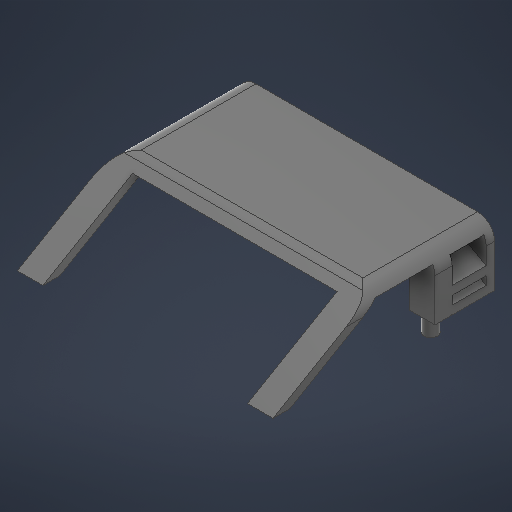
# Autodesk Inventor part: dach
Saved by Autodesk Inventor 2026.2 (Build 302298000, 298)
## iProperties
Created: 2026-08-16
Part Number: dach
Material: Tworzywo sztuczne ABS
Document SubType Name: Modeling
Designer: wojsl
Density: 1.06 g/cm^3
Appearance: Gładki — biały
Author: wojsl
Autodesk Inventor part; units mm, degrees
ref_plane "YZ Plane" through (0, 0, 0) normal (1, 0, 0) x (0, 1, 0)
ref_plane "XZ Plane" through (0, 0, 0) normal (0, 1, 0) x (-1, 0, 0)
ref_plane "XY Plane" through (0, 0, 0) normal (0, 0, 1) x (1, 0, 0)
sketch "Szkic1" plane through (0, 0, 0) normal (0, 0, 1) x (1, 0, 0)
  line L0 (-10.8101, 8.1046) -> (-12.3101, 8.1046)
  line L1 (-12.3101, 8.1046) -> (-12.3101, 11.6046)
  line L2 (-12.3101, 11.6046) -> (-10.8101, 11.6046)
  line L3 (-10.8101, 11.6046) -> (-10.8101, 8.1046)
  line L4 (-10.8101, 11.6046) -> (1.1899, 11.6046)
  line L5 (1.1899, 11.6046) -> (1.1899, 11.1716)
  line L6 (1.1899, 11.1716) -> (-10.8101, 11.1716)
  line L7 (-10.8101, 11.1716) -> (-10.8101, 11.6046)
  line L8 (1.1899, 11.6046) -> (2.6899, 11.6046)
  line L9 (2.6899, 11.6046) -> (2.6899, 8.1046)
  line L10 (2.6899, 8.1046) -> (1.1899, 8.1046)
  line L11 (1.1899, 8.1046) -> (1.1899, 11.6046)
  point P0 (0, 0)
  dimension "d0" = 1.5
  dimension "d1" = 1.5
  dimension "d2" = 15
  dimension "d3" = 0.433
  dimension "d6" = 3.5
  constraints: 24 end point, 6 parallel, 3 horizontal, 3 perpendicular, 1 point on line
  measures "d0" distance of L0.start L0.end
  measures "d1" distance of L9.end L10.end
  measures "d2" distance between parallel lines of L9 L1
  measures "d3" distance between parallel lines of L6 L4
  measures "d6" distance between parallel lines of L0 L4
extrude "Wyciągnięcie proste1" add sketch "Szkic1" along normal blind 13
sketch "Szkic2" plane through (-12.3101, 8.1046, 0) normal (-1, 0, 0) x (0, 0, 1)
  line L0 (0, 0) -> (13, 0) projected
  line L1 (13, 0) -> (7, 3.5)
  line L2 (0, 3.5) -> (13, 3.5) projected
  line L3 (0, 3.5) -> (0, 0) projected
  line L4 (13, 3.5) -> (13, 0) projected
  line L5 (13, 0) -> (13, 3.5)
  point P0 (0, -8.1046)
  dimension "d7" = 7
  constraints: 4 end point, 1 collinear, 1 point on line
  measures "d7" distance from line of L3 L1.end
extrude "Wyciągnięcie proste2" cut sketch "Szkic2" against normal through all contours L1 L2 L4
sketch "Szkic4" plane through (-12.3101, 8.1046, 0) normal (0, -1, 0) x (1, 0, 0)
  circle A0 centre (14.25, 3) radius 0.4
  line L0 (13.5, 0) -> (13.5, 13) projected
  line L1 (13.5, 0) -> (15, 0) projected
  circle A1 centre (0.75, 3) radius 0.4
  line L2 (0, 0) -> (1.5, 0) projected
  line L3 (0, 0) -> (0, 13) projected
  point P0 (12.3101, 0)
  dimension "d10" = 0.8
  dimension "d11" = 0.75
  dimension "d12" = 3
  dimension "d13" = 3
  dimension "d14" = 0.75
  dimension "d15" = 0.8
  constraints: 2 centre point
  measures "d10" diameter of A0
  measures "d11" distance from line of L0 A0.centre
  measures "d12" distance from line of L1 A0.centre
  measures "d13" distance from line of L2 A1.centre
  measures "d14" distance from line of L3 A1.centre
  measures "d15" diameter of A1
extrude "Wyciągnięcie proste3" add sketch "Szkic4" along normal blind 1
sketch "Szkic5" plane through (-12.3101, 8.1046, 0) normal (-1, 0, 0) x (0, 0, 1)
  line L0 (0, 0) -> (13, 0) projected
  line L1 (0, 3.5) -> (7, 3.5) projected
  line L2 (13, 0) -> (7, 3.5) projected
  line L3 (0, 3.5) -> (7, 3.5) projected
  line L4 (0, 3.5) -> (0, 0) projected
  line L5 (0, 0) -> (13, 0) projected
  line L6 (6.8648, 3) -> (11.1505, 0.5)
  line L7 (0.5, 0.5) -> (0.5, 3)
  line L8 (0.5, 3) -> (6.8648, 3)
  line L9 (11.1505, 0.5) -> (12.0077, 0)
  line L10 (0.5, 0.5) -> (0.5, 0)
  line L11 (2.5, 0) -> (2.5, 3)
  line L12 (3.5, 0) -> (3.5, 3)
  point P0 (0, -8.1046)
  dimension "d19" = 0.5
  dimension "d20" = 1
  dimension "d21" = 2
  constraints: 14 end point, 7 point on line, 3 perpendicular, 1 other
  measures "d19" distance between parallel lines of L2 L6
  measures "d20" distance between parallel lines of L11 L12
  measures "d21" distance between parallel lines of L7 L11
extrude "Wyciągnięcie proste4" cut sketch "Szkic5" against normal blind 15 contours L10 L7 L8 L11 L0 | L12 L8 L6 L9 L0
sketch "Szkic7" plane through (0, 0, 0) normal (0, 0, -1) x (-1, 0, 0)
  line L0 (12.3101, 11.6046) -> (12.3101, 8.1046) projected
  line L1 (12.3101, 8.1046) -> (10.8101, 8.9706)
  line L2 (10.8101, 8.1046) -> (10.8101, 11.1046) projected
  line L3 (12.3101, 8.6046) -> (10.8101, 9.4706)
  line L4 (12.3101, 8.1046) -> (10.8101, 8.1046) projected
  point P0 (0, 0)
  dimension "d33" = 60
  dimension "d34" = 60
  dimension "d35" = 0
  dimension "d36" = 0.5
  constraints: 4 end point, 4 point on line
  measures "d33" angle of L0 L3
  measures "d34" angle of L0 L1
  measures "d35" distance from line of L4 L1.start
  measures "d36" distance of L1.start L3.start
extrude "Wyciągnięcie proste6" add sketch "Szkic7" against normal blind 3 contours L0 L1 L2 L3
pattern_linear "Szyk prostokątny1" count 2 spacing 1 along (0, 1, 0) of "Wyciągnięcie proste6"
ref_plane "Płaszczyzna konstrukcyjna1" through (-4.8101, 8.1046, 0) normal (-1, 0, 0) x (0, 0, 1)
mirror "Odbij1" about plane through (-4.8101, 8.1046, 0) normal (-1, 0, 0) of "Wyciągnięcie proste6", "Szyk prostokątny1"
fillet "Zaokrąglenie1" radius 1 3 edges at (-12.3101, 11.6046, 3.5) (-4.8101, 11.6046, 7) (2.6899, 11.6046, 3.5)
